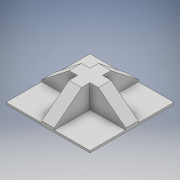
# Autodesk Inventor part: 障害物、山
Saved by Autodesk Inventor 2020 (Build 240168000, 168)
## iProperties
Part Number: 障害物、山
Material: 一般
Document SubType Name: Modeling
Designer: 雪村
Density: 1 g/cm^3
Appearance: 既定
Mass: 9453.75 g
Surface Area: 6917.12 cm^2
Volume: 9453.75 cm^3
Author: 雪村
Autodesk Inventor part; units mm, degrees
ref_plane "YZ Plane" through (0, 0, 0) normal (1, 0, 0) x (0, 1, 0)
ref_plane "XZ Plane" through (0, 0, 0) normal (0, 1, 0) x (-1, 0, 0)
ref_plane "XY Plane" through (0, 0, 0) normal (0, 0, 1) x (1, 0, 0)
sketch "スケッチ1" plane through (0, 0, 0) normal (0, 0, 1) x (1, 0, 0)
  line L0 (250, 250) -> (250, -250)
  line L1 (250, -250) -> (-250, -250)
  line L2 (-250, -250) -> (-250, 250)
  line L3 (-250, 250) -> (250, 250)
  point P0 (0, 0)
  point P1 (0, 0)
  dimension "d0" = 500
  constraints: 8 end point, 1 coincident, 1 horizontal, 9 other
  measures "d0" distance of L2.end L0.start
extrude "押し出し1" add sketch "スケッチ1" along normal blind 12
sketch "スケッチ2" plane through (0, 0, 12) normal (0, 0, 1) x (1, 0, 0)
  line L0 (250, -250) -> (250, 250) projected
  line L1 (250, 250) -> (-250, 250) projected
  line L2 (-250, 250) -> (-250, -250) projected
  line L3 (-250, -250) -> (250, -250) projected
  line L4 (-250, -250) -> (-37.5, -250)
  line L5 (-250, -250) -> (250, -250) projected
  line L6 (-37.5, -250) -> (37.5, -250)
  line L7 (-37.5, -250) -> (-37.5, 250)
  line L8 (37.5, -250) -> (37.5, 250)
  line L9 (250, 250) -> (-250, 250) projected
  line L10 (-250, -250) -> (-250, -37.5)
  line L11 (-250, 250) -> (-250, -250) projected
  line L12 (-250, -37.5) -> (250, -37.5)
  line L13 (-250, -37.5) -> (-250, 37.5)
  line L14 (-250, 37.5) -> (250, 37.5)
  point P0 (0, 0)
  dimension "d3" = 212.5
  dimension "d4" = 75
  dimension "d5" = 212.5
  dimension "d6" = 75
  constraints: 16 end point, 8 point on line, 2 horizontal, 2 vertical
  measures "d3" distance of L2.end L4.end
  measures "d4" distance of L4.end L6.end
  measures "d5" distance of L2.end L10.end
  measures "d6" distance of L10.end L13.end
extrude "押し出し2" add sketch "スケッチ2" along normal blind 10 contours L12 L8 L14 L0 | L3 L7 L12 L8 | L12 L7 L14 L8 | L14 L7 L1 L8 | L12 L2 L14 L7
sketch "スケッチ3" plane through (0, 0, 22) normal (0, 0, 1) x (1, 0, 0)
  line L0 (-37.5, -37.5) -> (-37.5, -250) projected
  line L1 (-37.5, -250) -> (37.5, -250) projected
  line L2 (37.5, -250) -> (37.5, -37.5) projected
  line L3 (37.5, -37.5) -> (250, -37.5) projected
  line L4 (250, -37.5) -> (250, 37.5) projected
  line L5 (250, 37.5) -> (37.5, 37.5) projected
  line L6 (37.5, 37.5) -> (37.5, 250) projected
  line L7 (37.5, 250) -> (-37.5, 250) projected
  line L8 (-37.5, 250) -> (-37.5, 37.5) projected
  line L9 (-37.5, 37.5) -> (-250, 37.5) projected
  line L10 (-250, 37.5) -> (-250, -37.5) projected
  line L11 (-250, -37.5) -> (-37.5, -37.5) projected
  point P0 (0, 0)
extrude "押し出し3" add sketch "スケッチ3" along normal blind 128
chamfer "面取り1" distance 162.5 distance2 128 1 edges at (-250, 0, 150) measured on face at (12.5, 179.1667, 150)
chamfer "面取り2" distance 162.5 distance2 128 1 edges at (0, -250, 150) measured on face at (12.5, 179.1667, 150)
chamfer "面取り3" distance 162.5 distance2 128 1 edges at (0, 250, 150) measured on face at (12.5, 108.3333, 150)
chamfer "面取り4" distance 162.5 distance2 128 1 edges at (250, 0, 150) measured on face at (108.3333, -12.5, 150)
sketch "スケッチ4" plane through (0, 0, 150) normal (0, 0, 1) x (1, 0, 0)
  circle A0 centre (0, 0) radius 0.005
  dimension "d23" = 0.01
  constraints: 1 centre point, 1 coincident
  measures "d23" diameter of A0
extrude "押し出し4" cut sketch "スケッチ4" against normal through all
